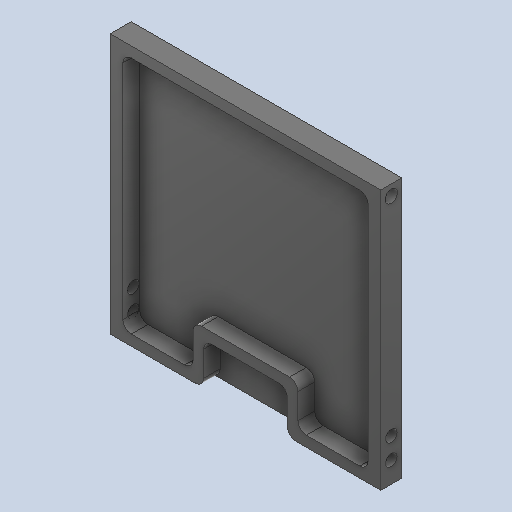
# Autodesk Inventor part: Cockpit_upper_back_door
Saved by Autodesk Inventor 2022.4 (Build 264492000, 492)
## iProperties
Created: 2021-11-08
Part Number: Cockpit_upper_back_door
Material: アセタール樹脂、黒
Document SubType Name: Modeling
Designer: Masato Kubotera
Density: 1.425 g/cm^3
Appearance: 滑らか - 黒
Mass: 9.62696 g
Surface Area: 104.205 cm^2
Volume: 6.75576 cm^3
Author: Masato Kubotera
Autodesk Inventor part; units mm, degrees
ref_plane "YZ Plane" through (0, 0, 0) normal (1, 0, 0) x (0, 1, 0)
ref_plane "XZ Plane" through (0, 0, 0) normal (0, 1, 0) x (-1, 0, 0)
ref_plane "XY Plane" through (0, 0, 0) normal (0, 0, 1) x (1, 0, 0)
sketch "スケッチ1" plane through (0, 0, 0) normal (0, 0, 1) x (1, 0, 0)
  line L0 (-32.25, 31) -> (32.25, 31)
  line L1 (32.25, 31) -> (32.25, -31)
  line L2 (32.25, -31) -> (10, -31)
  line L3 (-32.25, -31) -> (-32.25, 31)
  line L4 (-32.25, 31) -> (32.25, -31) construction
  line L5 (32.25, 31) -> (-32.25, -31) construction
  line L6 (-29.25, 28.5) -> (29.25, 28.5)
  line L7 (29.25, 28.5) -> (29.25, -28.5)
  line L8 (29.25, -28.5) -> (12.5, -28.5)
  line L9 (-29.25, -28.5) -> (-29.25, 28.5)
  line L10 (-29.25, 28.5) -> (29.25, -28.5) construction
  line L11 (29.25, 28.5) -> (-29.25, -28.5) construction
  line L12 (0, 31) -> (0, -28.25) construction
  line L13 (-10, -31) -> (-10, -21)
  line L14 (-10, -21) -> (10, -21)
  line L15 (10, -31) -> (10, -21)
  line L16 (-12.5, -28.5) -> (-12.5, -18.5)
  line L17 (-12.5, -18.5) -> (12.5, -18.5)
  line L18 (12.5, -28.5) -> (12.5, -18.5)
  line L19 (-12.5, -28.5) -> (-29.25, -28.5)
  line L20 (-10, -31) -> (-32.25, -31)
  line L21 (-10, -31) -> (10, -31)
  point P0 (0, 0)
  point P1 (10, -25.75)
  point P2 (10, -28.25)
  point P3 (-10, -25.75)
  dimension "d0" = 64.5
  dimension "d1" = 62
  dimension "d2" = 3
  dimension "d3" = 2.5
  dimension "d40" = 20
  dimension "d41" = 10
  dimension "d42" = 2.5
  dimension "d43" = 2.5
  constraints: 44 end point, 6 parallel, 5 midpoint, 4 perpendicular, 4 symmetric about line, 2 horizontal, 2 vertical, 1 collinear
  measures "d0" distance of L1.end L3.start
  measures "d1" distance of L0.end L1.end
  measures "d2" distance between parallel lines of L3 L9
  measures "d3" distance between parallel lines of L2 L8
  measures "d40" distance of L13.end L14.end
  measures "d41" distance of L13.start L13.end
  measures "d42" distance between parallel lines of L16 L13
  measures "d43" distance between parallel lines of L14 L17
extrude "押し出し1" add sketch "スケッチ1" along normal blind 5 contours L0 L1 L2 L15 L14 L13 L20 L3
extrude "押し出し2" add sketch "スケッチ1" along normal blind 1 contours L13 L14 L15 L21 | L6 L7 L8 L18 L17 L16 L19 L9
sketch "スケッチ2" plane through (32.25, -31, 0) normal (1, 0, 0) x (0, 0, -1)
  line L0 (0, 0) -> (-5, 0) projected
  line L1 (0, 62) -> (-5, 62) projected
  line L2 (-2.5, 62) -> (-2.5, 0) construction
  point P0 (0, 31)
  point P1 (-2.5, 59.5)
  point P2 (-2.5, 5)
  point P3 (-2.5, 10)
  dimension "d8" = 5
  dimension "d9" = 5
  dimension "d10" = 2.5
  constraints: 3 point on line, 2 end point, 2 midpoint
  measures "d8" distance from line of L0 point (-2.5, 5)
  measures "d9" distance of point (-2.5, 5) point (-2.5, 10)
  measures "d10" distance from line of point (-2.5, 59.5) L1
hole "穴1" at (32.25, 28.5, 2.5) direction (-1, 0, 0) diameter 3 depth 2.9
hole "穴2" at (32.25, -21, 2.5) at (32.25, -26, 2.5) direction (-1, 0, 0) diameter 2.8 depth 3
fillet "フィレット1" radius 2 12 edges at (-29.25, 28.5, 3) (29.25, -28.5, 3) (29.25, 28.5, 3) (-12.5, -28.5, 3) (-29.25, -28.5, 3) (12.5, -28.5, 3) (10, -21, 3) (-10, -21, 3) (-12.5, -18.5, 3) (12.5, -18.5, 3) (-10, -31, 3) (10, -31, 3)
sketch "スケッチ3" plane through (-32.25, -31, 0) normal (-1, 0, 0) x (0, 0, 1)
  circle A0 centre (2.5, 59.5) radius 1.5 projected
  arc A1 (3.8077, 4.5) -> (1.1923, 4.5) centre (2.5, 5) ccw projected
  circle A2 centre (2.5, 10) radius 1.4 projected
  point P0 (0, 31)
  point P1 (2.5, 5)
  point P2 (2.5, 10)
  constraints: 3 coincident
hole "穴3" at (-32.25, 28.5, 2.5) direction (1, 0, 0) diameter 3 depth 2.9
hole "穴4" at (-32.25, -26, 2.5) at (-32.25, -21, 2.5) direction (1, 0, 0) diameter 2.8 depth 3
equation "\"d43\" = d42"
